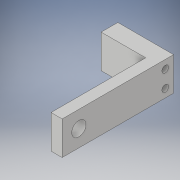
# Autodesk Inventor part: PaddleCollection2.1WheelBracket
Saved by Autodesk Inventor 2019 (Build 230136000, 136)
## iProperties
Created: 2018-10-27
Part Number: PaddleCollection2.1WheelBracket
Material: Generic
Document SubType Name: Modeling
Designer: User
Density: 1 g/cm^3
Appearance: Default
Author: User
Autodesk Inventor part; units mm, degrees
ref_plane "YZ Plane" through (0, 0, 0) normal (1, 0, 0) x (0, 1, 0)
ref_plane "XZ Plane" through (0, 0, 0) normal (0, 1, 0) x (-1, 0, 0)
ref_plane "XY Plane" through (0, 0, 0) normal (0, 0, 1) x (1, 0, 0)
sketch "Sketch1" plane through (0, 0, 0) normal (0, 1, 0) x (-1, 0, 0)
  line L0 (0, 0) -> (-31.75, 0)
  line L1 (-31.75, 0) -> (-31.75, 63.5)
  line L2 (-31.75, 63.5) -> (0, 63.5)
  line L3 (0, 63.5) -> (0, 0)
  line L4 (0, 63.5) -> (-25.4, 63.5)
  line L5 (-25.4, 63.5) -> (-25.4, 9.525)
  line L6 (-25.4, 9.525) -> (0, 9.525)
  line L7 (0, 9.525) -> (0, 63.5)
  dimension "d0" = 63.5
  dimension "d1" = 31.75
  dimension "d2" = 9.525
  dimension "d3" = 6.35
  constraints: 16 end point, 4 parallel, 2 horizontal, 2 perpendicular
  measures "d0" distance of L0.end L1.end
  measures "d1" distance of L1.end L2.end
  measures "d2" distance between parallel lines of L0 L6
  measures "d3" distance between parallel lines of L1 L5
extrude "Extrusion1" add sketch "Sketch1" along normal blind 19.05 contours L0 L1 L2 L5 L6 L3
sketch "Sketch2" plane through (31.75, 0, 63.5) normal (1, 0, 0) x (0, 0, -1)
  line L0 (0, 0) -> (63.5, 0) projected
  line L1 (63.5, 0) -> (63.5, 19.05) projected
  line L2 (0, 19.05) -> (63.5, 19.05) projected
  line L3 (0, 0) -> (0, 19.05) projected
  point P0 (9.525, 9.525)
  dimension "d6" = 19.05
  dimension "d7" = 9.525
  dimension "d8" = 9.525
  measures "d6" distance of L0.start L2.start
  measures "d7" distance from line of L2 point (9.525, 9.525)
  measures "d8" distance from line of L3 point (9.525, 9.525)
hole "Hole1" at (31.75, 9.525, 53.975) direction (-1, 0, 0) diameter 8.128 depth 10.9728 tip angle 118
sketch "Sketch3" plane through (0, 0, 0) normal (-1, 0, 0) x (0, 0, 1)
  line L0 (9.525, 0) -> (9.525, 19.05) projected
  line L1 (0, 19.05) -> (9.525, 19.05) projected
  line L2 (0, 0) -> (0, 19.05) projected
  line L3 (0, 0) -> (9.525, 0) projected
  point P0 (4.7625, 4.7625)
  point P1 (4.7625, 14.2875)
  dimension "d16" = 9.525
  dimension "d17" = 9.525
  dimension "d18" = 4.7625
  dimension "d19" = 19.05
  dimension "d20" = 4.7625
  dimension "d21" = 4.7625
  measures "d16" distance of point (4.763, 14.288) point (4.763, 4.763)
  measures "d17" distance of L2.start L0.start
  measures "d18" distance from line of L2 point (4.763, 4.763)
  measures "d19" distance of L2.start L1.start
  measures "d20" distance from line of L3 point (4.763, 4.763)
  measures "d21" distance from line of L2 point (4.763, 14.288)
hole "Hole2" at (0, 4.7625, 4.7625) at (0, 14.2875, 4.7625) direction (1, 0, 0) diameter 3.81 end through all
equation "\"d7\" = 0.5 * d6"
equation "\"d8\" = d7"
equation "\"d18\" = 0.5 * d17"
equation "\"d20\" = -0.5 * d16 + 0.5 * d19"
equation "\"d21\" = d18"
body "Solid1"
